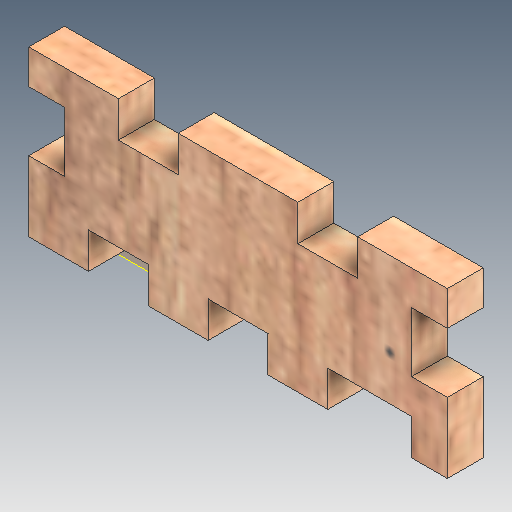
# Autodesk Inventor part: onderzijde joystickdoosje
Saved by Autodesk Inventor 2020.3 (Build 243373000, 373)
## iProperties
Created: 2020-12-09
Part Number: onderzijde joystickdoosje
Material: Wood (Birch)
Document SubType Name: Sheet Metal
Designer: Svend
Density: 0.55 g/cm^3
Sheet Metal Rule: Default_mm
Appearance: Birch - Natural Polished
Author: Svend
Autodesk Inventor part; units mm, degrees
ref_plane "YZ Plane" through (0, 0, 0) normal (1, 0, 0) x (0, 1, 0)
ref_plane "XZ Plane" through (0, 0, 0) normal (0, 1, 0) x (-1, 0, 0)
ref_plane "XY Plane" through (0, 0, 0) normal (0, 0, 1) x (1, 0, 0)
ref_plane "Work Plane1" through (-10.7838, -0.756, 0) normal (0, 0, 1) x (1, 0, 0)
sketch "Sketch1" plane through (-10.7838, -0.756, 0) normal (0, 0, 1) x (1, 0, 0)
  line L0 (-33.2162, 0.756) -> (-33.2162, 6.756)
  line L1 (-33.2162, 0.756) -> (-23.2162, 0.756)
  line L2 (-23.2162, 0.756) -> (-23.2162, 6.756)
  line L3 (-23.2162, 6.756) -> (-33.2162, 6.756)
  line L4 (-3.2162, 0.756) -> (-3.2162, 6.756)
  line L5 (-3.2162, 6.756) -> (-13.2162, 6.756)
  line L6 (-13.2162, 0.756) -> (-13.2162, 6.756)
  line L7 (-13.2162, 0.756) -> (-3.2162, 0.756)
  line L8 (-135.7005, 28.256) -> (83.2995, 28.256)
  line L9 (83.2995, 43.256) -> (-135.7005, 43.256)
  line L10 (-43.2162, 0.756) -> (-43.2162, 6.756)
  line L11 (-43.2162, 6.756) -> (-47.2162, 6.756)
  line L12 (-47.2162, 0.756) -> (-47.2162, 6.756)
  line L13 (-47.2162, 0.756) -> (-43.2162, 0.756)
  line L14 (16.7838, 6.756) -> (10.7838, 6.756)
  line L15 (10.7838, 0.756) -> (10.7838, 6.756)
  line L16 (10.7838, 0.756) -> (16.7838, 0.756)
  line L17 (16.7838, 0.756) -> (16.7838, 6.756)
  line L18 (-53.2162, 6.756) -> (-53.2162, 0.756)
  line L19 (-47.2162, 0.756) -> (-53.2162, 0.756)
  line L20 (-47.2162, 0.756) -> (-47.2162, 6.756)
  line L21 (-47.2162, 6.756) -> (-53.2162, 6.756)
  line L22 (-53.2162, 6.756) -> (16.7838, 6.756)
  line L23 (16.7838, 6.756) -> (16.7838, 28.256)
  line L24 (16.7838, 28.256) -> (-53.2162, 28.256)
  line L25 (-53.2162, 28.256) -> (-53.2162, 6.756)
  line L26 (-53.2162, 12.506) -> (-47.2162, 12.506)
  line L27 (-47.2162, 12.506) -> (-47.2162, 22.506)
  line L28 (-47.2162, 22.506) -> (-53.2162, 22.506)
  line L29 (-53.2162, 22.506) -> (-53.2162, 12.506)
  line L30 (16.7838, 22.506) -> (10.7838, 22.506)
  line L31 (10.7838, 22.506) -> (10.7838, 12.506)
  line L32 (10.7838, 12.506) -> (16.7838, 12.506)
  line L33 (16.7838, 12.506) -> (16.7838, 22.506)
  line L34 (-38.2162, 28.256) -> (-28.2162, 28.256)
  line L35 (-28.2162, 28.256) -> (-28.2162, 22.256)
  line L36 (-28.2162, 22.256) -> (-38.2162, 22.256)
  line L37 (-38.2162, 22.256) -> (-38.2162, 28.256)
  line L38 (1.7838, 28.256) -> (-8.2162, 28.256)
  line L39 (-8.2162, 28.256) -> (-8.2162, 22.256)
  line L40 (-8.2162, 22.256) -> (1.7838, 22.256)
  line L41 (1.7838, 22.256) -> (1.7838, 28.256)
  point P0 (-47.2162, 17.506)
  point P1 (-53.2162, 17.506)
  point P2 (10.7838, 17.506)
  point P3 (16.7838, 17.506)
extrude "Plate1" add sketch "Sketch1" along normal blind 6 contours L0 L3 L2 L1 | L22 L11 L21 L25 L26 L27 L28 L8 L37 L36 L35 L39 L40 L41 L23 L30 L31 L32 L14 L5 L3 | L10 L13 L12 L11 | L5 L4 L7 L6 | L12 L19 L18 L21 | L14 L17 L16 L15
equation "\"d10\" = Thickness"
equation "\"BendRadius\" = Thickness"
equation "\"BendReliefWidth\" = Thickness"
equation "\"BendReliefDepth\" = 0.5 * Thickness"
equation "\"CornerReliefSize\" = 4 * Thickness"
equation "\"MinimumRemnant\" = 2 * Thickness"
equation "\"TransitionRadius\" = BendRadius"
equation "\"JacobiRadiusSize\" = BendRadius"
equation "\"GapSize\" = Thickness"
equation "\"d9\" = d8"
equation "\"Thickness\" = 6"
equation "\"d8\" = 15"
body "Solid1"
